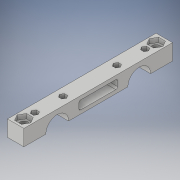
# Autodesk Inventor part: Mount_Block
Saved by Autodesk Inventor 2019 (Build 230136000, 136)
## iProperties
Created: 2019-10-21
Part Number: Mount_Block
Material: Generic
Document SubType Name: Modeling
Designer: 19879326
Density: 1 g/cm^3
Appearance: Default
Author: 19879326
Autodesk Inventor part; units mm, degrees
ref_plane "YZ Plane" through (0, 0, 0) normal (1, 0, 0) x (0, 1, 0)
ref_plane "XZ Plane" through (0, 0, 0) normal (0, 1, 0) x (-1, 0, 0)
ref_plane "XY Plane" through (0, 0, 0) normal (0, 0, 1) x (1, 0, 0)
sketch "Sketch1" plane through (0, 0, 0) normal (1, 0, 0) x (0, 1, 0)
  arc A0 (0, 32.5) -> (0, 57.5) centre (0, 45) ccw
  arc A1 (0, -57.5) -> (0, -32.5) centre (0, -45) ccw
  line L0 (0, 81.5) -> (17.5, 81.5)
  line L1 (17.5, 81.5) -> (17.5, -81.5)
  line L2 (17.5, -81.5) -> (0, -81.5)
  line L3 (0, 57.5) -> (0, 81.5)
  line L4 (0, -81.5) -> (0, -57.5)
  line L5 (0, -32.5) -> (0, 32.5)
  point P0 (0, 0)
  point P1 (0, 0)
  point P2 (17.5, 0)
  point P3 (0, 69.5)
  point P4 (0, -69.5)
  point P5 (12.5, 45)
  dimension "d0" = 25
  dimension "d2" = 90
  dimension "d3" = 45
  dimension "d4" = 24
  dimension "d15" = 5
  constraints: 12 end point, 5 point on circle, 4 midpoint, 4 parallel, 3 vertical alignment, 2 centre point, 2 coincident, 1 equal radius, 1 horizontal, 1 horizontal alignment, 1 perpendicular
  measures "d0" diameter of A0
  measures "d2" distance of A1.centre A0.centre
  measures "d3" distance of point (0, 0) A1.centre
  measures "d4" distance from line of L0 L3.start
  measures "d15" distance from line of L1 point (12.5, 45)
extrude "Extrusion1" add sketch "Sketch1" along normal blind 18
sketch "Sketch2" plane through (0, 17.5, 81.5) normal (0, 1, 0) x (1, 0, 0)
  circle A0 centre (9, 9) radius 4.35
  circle A1 centre (9, 154) radius 4.35
  line L0 (18, 163) -> (18, 0) projected
  line L1 (0, 0) -> (18, 0) projected
  line L2 (0, 163) -> (18, 163) projected
  point P0 (0, 81.5)
  dimension "d7" = 8.7
  dimension "d8" = 8.7
  dimension "d9" = 9
  dimension "d10" = 9
  dimension "d11" = 9
  constraints: 2 centre point, 1 vertical alignment
  measures "d7" diameter of A0
  measures "d8" diameter of A1
  measures "d9" distance from line of L0 A0.centre
  measures "d10" distance from line of A0.centre L1
  measures "d11" distance from line of L2 A1.centre
extrude "Extrusion2" cut sketch "Sketch2" against normal blind 29.5
sketch "Sketch3" plane through (0, 17.5, 81.5) normal (0, 1, 0) x (1, 0, 0)
  circle A0 centre (9, 154) radius 4.35 projected
  line L0 (12.7528, 160.5) -> (16.5056, 154)
  line L1 (16.5056, 154) -> (12.7528, 147.5)
  line L2 (12.7528, 147.5) -> (5.2472, 147.5)
  line L3 (5.2472, 147.5) -> (1.4944, 154)
  line L4 (1.4944, 154) -> (5.2472, 160.5)
  line L5 (5.2472, 160.5) -> (12.7528, 160.5)
  line L6 (0, 163) -> (18, 163) projected
  circle A1 centre (9, 9) radius 4.35 projected
  line L7 (12.7528, 2.5) -> (5.2472, 2.5)
  line L8 (5.2472, 2.5) -> (1.4944, 9)
  line L9 (1.4944, 9) -> (5.2472, 15.5)
  line L10 (5.2472, 15.5) -> (12.7528, 15.5)
  line L11 (12.7528, 15.5) -> (16.5056, 9)
  line L12 (16.5056, 9) -> (12.7528, 2.5)
  line L13 (0, 0) -> (18, 0) projected
  point P0 (0, 81.5)
  dimension "d16" = 13
  dimension "d17" = 13
  constraints: 24 end point, 2 coincident, 2 parallel, 26 other
  measures "d16" distance between parallel lines of L2 L5
  measures "d17" distance between parallel lines of L10 L7
extrude "Extrusion3" cut sketch "Sketch3" against normal blind 5
sketch "Sketch4" plane through (0, 0, 57.5) normal (0, -1, 0) x (1, 0, 0)
  circle A0 centre (9, 3) radius 1.5
  circle A1 centre (9, -28) radius 1.5
  circle A2 centre (9, -87) radius 1.5
  circle A3 centre (9, -118) radius 1.5
  line L0 (0, 0) -> (18, 0) projected
  line L1 (0, -25) -> (18, -25) projected
  line L2 (0, -90) -> (18, -90) projected
  line L3 (0, -115) -> (18, -115) projected
  line L4 (0, -139) -> (18, -139) projected
  point P0 (0, -57.5)
  point P1 (9, -139)
  dimension "d20" = 3
  dimension "d21" = 3
  dimension "d22" = 3
  dimension "d23" = 3
  dimension "d24" = 3
  constraints: 4 centre point, 4 vertical alignment, 3 equal radius, 1 midpoint
  measures "d20" diameter of A0
  measures "d21" distance from line of L0 A0.centre
  measures "d22" distance from line of L1 A1.centre
  measures "d23" distance from line of L2 A2.centre
  measures "d24" distance from line of A3.centre L3
extrude "Extrusion4" cut sketch "Sketch4" against normal blind 22
sketch "Sketch5" plane through (0, 17.5, 81.5) normal (0, 1, 0) x (1, 0, 0)
  circle A0 centre (9, 21) radius 1.5 projected
  line L0 (10.8764, 24.25) -> (12.7528, 21)
  line L1 (12.7528, 21) -> (10.8764, 17.75)
  line L2 (10.8764, 17.75) -> (7.1236, 17.75)
  line L3 (7.1236, 17.75) -> (5.2472, 21)
  line L4 (5.2472, 21) -> (7.1236, 24.25)
  line L5 (7.1236, 24.25) -> (10.8764, 24.25)
  circle A1 centre (9, 52) radius 1.5 projected
  line L6 (7.1236, 55.25) -> (10.8764, 55.25)
  line L7 (10.8764, 55.25) -> (12.7528, 52)
  line L8 (12.7528, 52) -> (10.8764, 48.75)
  line L9 (10.8764, 48.75) -> (7.1236, 48.75)
  line L10 (7.1236, 48.75) -> (5.2472, 52)
  line L11 (5.2472, 52) -> (7.1236, 55.25)
  circle A2 centre (9, 111) radius 1.5 projected
  line L12 (7.1236, 114.25) -> (10.8764, 114.25)
  line L13 (10.8764, 114.25) -> (12.7528, 111)
  line L14 (12.7528, 111) -> (10.8764, 107.75)
  line L15 (10.8764, 107.75) -> (7.1236, 107.75)
  line L16 (7.1236, 107.75) -> (5.2472, 111)
  line L17 (5.2472, 111) -> (7.1236, 114.25)
  circle A3 centre (9, 142) radius 1.5 projected
  line L18 (7.1236, 145.25) -> (10.8764, 145.25)
  line L19 (10.8764, 145.25) -> (12.7528, 142)
  line L20 (12.7528, 142) -> (10.8764, 138.75)
  line L21 (10.8764, 138.75) -> (7.1236, 138.75)
  line L22 (7.1236, 138.75) -> (5.2472, 142)
  line L23 (5.2472, 142) -> (7.1236, 145.25)
  line L24 (12.7528, 147.5) -> (5.2472, 147.5) projected
  point P0 (0, 81.5)
  dimension "d27" = 6.5
  dimension "d28" = 6.5
  dimension "d29" = 6.5
  dimension "d30" = 6.5
  constraints: 48 end point, 4 coincident, 4 parallel, 52 other
  measures "d27" distance between parallel lines of L5 L2
  measures "d28" distance between parallel lines of L6 L9
  measures "d29" distance between parallel lines of L12 L15
  measures "d30" distance between parallel lines of L18 L21
extrude "Extrusion5" cut sketch "Sketch5" against normal blind 7.5
sketch "Sketch6" plane through (18, 0, 0) normal (1, 0, 0) x (0, 0, -1)
  line L0 (-21.25, 13.5) -> (21.25, 13.5)
  line L1 (21.25, 13.5) -> (21.25, 4)
  line L2 (21.25, 4) -> (-21.25, 4)
  line L3 (-21.25, 4) -> (-21.25, 13.5)
  line L4 (-26.25, 17.5) -> (-26.25, 10) projected
  line L5 (26.25, 17.5) -> (26.25, 10) projected
  line L6 (81.5, 17.5) -> (-81.5, 17.5) projected
  point P0 (0, 0)
  dimension "d33" = 5
  dimension "d34" = 5
  dimension "d35" = 4
  dimension "d36" = 4
  constraints: 8 end point, 2 parallel, 1 horizontal, 1 perpendicular
  measures "d33" distance between parallel lines of L3 L4
  measures "d34" distance between parallel lines of L5 L1
  measures "d35" distance between parallel lines of L6 L0
  measures "d36" distance from line of point (0, 0) L2
extrude "Extrusion6" cut sketch "Sketch6" against normal blind 60.25
fillet "Fillet1" radius 2 4 edges at (9, 4, 21.25) (9, 13.5, 21.25) (9, 13.5, -21.25) (9, 4, -21.25)
body "Solid1"
